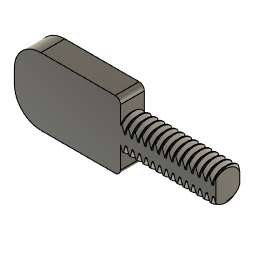
Printable 14-20 Bolt Handle v1 (Autodesk Fusion 360 design; units mm, degrees)
Autodesk Fusion 360 part; units mm, degrees
sketch "Sketch1" plane through (0, 0, 0) normal (1, 0, 0) x (0, 1, 0)
  circle A0 centre (0, 0) radius 3.175
  dimension "d1" = 6.35
  constraint coincident A0.centre origin
  measures "d1" diameter of A0
extrude "Extrude1" add sketch "Sketch1" along normal blind 18
sketch "Sketch2" plane through (0, 0, 0) normal (-1, 0, 0) x (0, -1, 0)
  circle A0 centre (0, 0) radius 3.175
  line L0 (5.5, 3.1754) -> (0, 6.3509)
  line L1 (0, 6.3509) -> (-5.5, 3.1754)
  line L2 (-5.5, 3.1754) -> (-5.5, -3.1754)
  line L3 (-5.5, -3.1754) -> (0, -6.3509)
  line L4 (0, -6.3509) -> (5.5, -3.1754)
  line L5 (5.5, -3.1754) -> (5.5, 3.1754)
  dimension "d4" = 11
  constraint coincident A0.centre origin
  constraint vertical L5
  measures "d4" distance of L2 L5
extrude "Extrude2" add sketch "Sketch2" along normal blind 4 contours A0 | L0 L1 L2 L3 L4 L5
thread "Thread1" "ANSI Unified Screw Threads 0.25 1/4-20 UNC 3A" major diameter 6.2484 minor diameter 4.8387 pitch 1.27 angle 60 modelled right hand crest width 0.1965 on face at (12, 3.1711, -0.1583) crest through (-0.3175, 3.1242, 0)
sketch "Sketch3" plane through (-4, 0, 0) normal (-1, 0, 0) x (0, -1, 0)
  line L0 (5.5, -3.1754) -> (5.5, 3.1754)
  line L1 (5.5, 3.1754) -> (0, 6.3509)
  line L2 (0, 6.3509) -> (-5.5, 3.1754)
  line L3 (-5.5, 3.1754) -> (-5.5, -3.1754)
  line L4 (-5.5, -3.1754) -> (0, -6.3509)
  line L5 (0, -6.3509) -> (5.5, -3.1754)
  line L6 (0, 0) -> (0, 21) construction
  line L7 (0, 0) -> (0, -19) construction
  line L8 (2.25, 5.0518) -> (2.25, -5.0518)
  line L9 (-2.25, 5.0518) -> (-2.25, -5.0518)
  dimension "d7" = 2.25
  dimension "d8" = 2.25
  constraint coincident L6.start L7.start
  constraint parallel L0 L6
  constraint parallel L6 L7
  constraint coincident L1 L8.start
  constraint coincident L5 L8.end
  constraint parallel L6 L8
  constraint coincident L2 L9.start
  constraint coincident L4 L9.end
  constraint parallel L7 L9
  measures "d7" distance of L6.start L9
  measures "d8" distance of L6 L8
extrude "Extrude3" cut sketch "Sketch3" against normal through all contours L0 L1 L5 L8 | L2 L3 L4 L9
sketch "Sketch4" plane through (0, -2.25, 0) normal (0, -1, 0) x (1, 0, 0)
  line L0 (0, -5.0518) -> (0, -1.2384)
  spline S0 degree 3 poles (0.3742, -2.1675) (0.295, -1.9904) (0.2175, -1.8092) (0.0949, -1.5007) (0.0458, -1.3702) (0, -1.2384) knots -0.136565 -0.136565 -0.136565 -0.136565 -0.077979 -0.077979 -0.036476 -0.036476 -0.036476 -0.036476
  line L1 (0.3742, -2.1675) -> (0.5707, -2.1675)
  spline S1 degree 3 poles (0.8988, -0.8892) (0.8665, -1.1289) (0.8148, -1.3659) (0.6999, -1.784) (0.6406, -1.969) (0.5748, -2.1561) (0.5728, -2.1618) (0.5707, -2.1675) knots -0.131697 -0.131697 -0.131697 -0.131697 -0.059487 -0.059487 -0.001818 -0.001818 0 0 0 0
  line L2 (0.8988, -0.8892) -> (1.1584, -0.8892)
  spline S2 degree 3 poles (1.6442, -2.1675) (1.565, -1.9904) (1.4875, -1.8092) (1.3222, -1.3933) (1.2345, -1.1492) (1.1614, -0.8997) (1.1599, -0.8945) (1.1584, -0.8892) knots -0.136565 -0.136565 -0.136565 -0.136565 -0.077979 -0.077979 -0.001638 -0.001638 0 0 0 0
  line L3 (1.6442, -2.1675) -> (1.8407, -2.1675)
  spline S3 degree 3 poles (2.1688, -0.8892) (2.1365, -1.1289) (2.0848, -1.3659) (1.9699, -1.784) (1.9106, -1.969) (1.8448, -2.1561) (1.8428, -2.1618) (1.8407, -2.1675) knots -0.131697 -0.131697 -0.131697 -0.131697 -0.059487 -0.059487 -0.001818 -0.001818 0 0 0 0
  line L4 (2.1688, -0.8892) -> (2.4284, -0.8892)
  spline S4 degree 3 poles (2.9142, -2.1675) (2.835, -1.9904) (2.7575, -1.8092) (2.5922, -1.3933) (2.5045, -1.1492) (2.4314, -0.8997) (2.4299, -0.8945) (2.4284, -0.8892) knots -0.136565 -0.136565 -0.136565 -0.136565 -0.077979 -0.077979 -0.001638 -0.001638 0 0 0 0
  line L5 (2.9142, -2.1675) -> (3.1107, -2.1675)
  spline S5 degree 3 poles (3.4388, -0.8892) (3.4065, -1.1289) (3.3548, -1.3659) (3.2399, -1.784) (3.1806, -1.969) (3.1148, -2.1561) (3.1128, -2.1618) (3.1107, -2.1675) knots -0.131697 -0.131697 -0.131697 -0.131697 -0.059487 -0.059487 -0.001818 -0.001818 0 0 0 0
  line L6 (3.4388, -0.8892) -> (3.6984, -0.8892)
  spline S6 degree 3 poles (4.1842, -2.1675) (4.105, -1.9904) (4.0275, -1.8092) (3.8622, -1.3933) (3.7745, -1.1492) (3.7014, -0.8997) (3.6999, -0.8945) (3.6984, -0.8892) knots -0.136565 -0.136565 -0.136565 -0.136565 -0.077979 -0.077979 -0.001638 -0.001638 0 0 0 0
  line L7 (4.1842, -2.1675) -> (4.3807, -2.1675)
  spline S7 degree 3 poles (4.7088, -0.8892) (4.6765, -1.1289) (4.6248, -1.3659) (4.5099, -1.784) (4.4506, -1.969) (4.3848, -2.1561) (4.3828, -2.1618) (4.3807, -2.1675) knots -0.131697 -0.131697 -0.131697 -0.131697 -0.059487 -0.059487 -0.001818 -0.001818 0 0 0 0
  line L8 (4.7088, -0.8892) -> (4.9684, -0.8892)
  spline S8 degree 3 poles (5.4542, -2.1675) (5.375, -1.9904) (5.2975, -1.8092) (5.1322, -1.3933) (5.0445, -1.1492) (4.9714, -0.8997) (4.9699, -0.8945) (4.9684, -0.8892) knots -0.136565 -0.136565 -0.136565 -0.136565 -0.077979 -0.077979 -0.001638 -0.001638 0 0 0 0
  line L9 (5.4542, -2.1675) -> (5.6507, -2.1675)
  spline S9 degree 3 poles (5.9788, -0.8892) (5.9465, -1.1289) (5.8948, -1.3659) (5.7799, -1.784) (5.7206, -1.969) (5.6548, -2.1561) (5.6528, -2.1618) (5.6507, -2.1675) knots -0.131697 -0.131697 -0.131697 -0.131697 -0.059487 -0.059487 -0.001818 -0.001818 0 0 0 0
  line L10 (5.9788, -0.8892) -> (6.2384, -0.8892)
  spline S10 degree 3 poles (6.7242, -2.1675) (6.645, -1.9904) (6.5675, -1.8092) (6.4022, -1.3933) (6.3145, -1.1492) (6.2414, -0.8997) (6.2399, -0.8945) (6.2384, -0.8892) knots -0.136565 -0.136565 -0.136565 -0.136565 -0.077979 -0.077979 -0.001638 -0.001638 0 0 0 0
  line L11 (6.7242, -2.1675) -> (6.9207, -2.1675)
  spline S11 degree 3 poles (7.2488, -0.8892) (7.2165, -1.1289) (7.1648, -1.3659) (7.0499, -1.784) (6.9906, -1.969) (6.9248, -2.1561) (6.9228, -2.1618) (6.9207, -2.1675) knots -0.131697 -0.131697 -0.131697 -0.131697 -0.059487 -0.059487 -0.001818 -0.001818 0 0 0 0
  line L12 (7.2488, -0.8892) -> (7.5084, -0.8892)
  spline S12 degree 3 poles (7.9942, -2.1675) (7.915, -1.9904) (7.8375, -1.8092) (7.6722, -1.3933) (7.5845, -1.1492) (7.5114, -0.8997) (7.5099, -0.8945) (7.5084, -0.8892) knots -0.136565 -0.136565 -0.136565 -0.136565 -0.077979 -0.077979 -0.001638 -0.001638 0 0 0 0
  line L13 (7.9942, -2.1675) -> (8.1907, -2.1675)
  spline S13 degree 3 poles (8.5188, -0.8892) (8.4865, -1.1289) (8.4348, -1.3659) (8.3199, -1.784) (8.2606, -1.969) (8.1948, -2.1561) (8.1928, -2.1618) (8.1907, -2.1675) knots -0.131697 -0.131697 -0.131697 -0.131697 -0.059487 -0.059487 -0.001818 -0.001818 0 0 0 0
  line L14 (8.5188, -0.8892) -> (8.7784, -0.8892)
  spline S14 degree 3 poles (9.2642, -2.1675) (9.185, -1.9904) (9.1075, -1.8092) (8.9422, -1.3933) (8.8545, -1.1492) (8.7814, -0.8997) (8.7799, -0.8945) (8.7784, -0.8892) knots -0.136565 -0.136565 -0.136565 -0.136565 -0.077979 -0.077979 -0.001638 -0.001638 0 0 0 0
  line L15 (9.2642, -2.1675) -> (9.4607, -2.1675)
  spline S15 degree 3 poles (9.7888, -0.8892) (9.7565, -1.1289) (9.7048, -1.3659) (9.5899, -1.784) (9.5306, -1.969) (9.4648, -2.1561) (9.4628, -2.1618) (9.4607, -2.1675) knots -0.131697 -0.131697 -0.131697 -0.131697 -0.059487 -0.059487 -0.001818 -0.001818 0 0 0 0
  line L16 (9.7888, -0.8892) -> (10.0484, -0.8892)
  spline S16 degree 3 poles (10.5342, -2.1675) (10.455, -1.9904) (10.3775, -1.8092) (10.2122, -1.3933) (10.1245, -1.1492) (10.0514, -0.8997) (10.0499, -0.8945) (10.0484, -0.8892) knots -0.136565 -0.136565 -0.136565 -0.136565 -0.077979 -0.077979 -0.001638 -0.001638 0 0 0 0
  line L17 (10.5342, -2.1675) -> (10.7307, -2.1675)
  spline S17 degree 3 poles (11.0588, -0.8892) (11.0265, -1.1289) (10.9748, -1.3659) (10.8599, -1.784) (10.8006, -1.969) (10.7348, -2.1561) (10.7328, -2.1618) (10.7307, -2.1675) knots -0.131697 -0.131697 -0.131697 -0.131697 -0.059487 -0.059487 -0.001818 -0.001818 0 0 0 0
  line L18 (11.0588, -0.8892) -> (11.3184, -0.8892)
  spline S18 degree 3 poles (11.8042, -2.1675) (11.725, -1.9904) (11.6475, -1.8092) (11.4822, -1.3933) (11.3945, -1.1492) (11.3214, -0.8997) (11.3199, -0.8945) (11.3184, -0.8892) knots -0.136565 -0.136565 -0.136565 -0.136565 -0.077979 -0.077979 -0.001638 -0.001638 0 0 0 0
  line L19 (11.8042, -2.1675) -> (12.0007, -2.1675)
  spline S19 degree 3 poles (12.3288, -0.8892) (12.2965, -1.1289) (12.2448, -1.3659) (12.1299, -1.784) (12.0706, -1.969) (12.0048, -2.1561) (12.0028, -2.1618) (12.0007, -2.1675) knots -0.131697 -0.131697 -0.131697 -0.131697 -0.059487 -0.059487 -0.001818 -0.001818 0 0 0 0
  line L20 (12.3288, -0.8892) -> (12.5884, -0.8892)
  spline S20 degree 3 poles (13.0742, -2.1675) (12.995, -1.9904) (12.9175, -1.8092) (12.7522, -1.3933) (12.6645, -1.1492) (12.5914, -0.8997) (12.5899, -0.8945) (12.5884, -0.8892) knots -0.136565 -0.136565 -0.136565 -0.136565 -0.077979 -0.077979 -0.001638 -0.001638 0 0 0 0
  line L21 (13.0742, -2.1675) -> (13.2707, -2.1675)
  spline S21 degree 3 poles (13.5988, -0.8892) (13.5665, -1.1289) (13.5148, -1.3659) (13.3999, -1.784) (13.3406, -1.969) (13.2748, -2.1561) (13.2728, -2.1618) (13.2707, -2.1675) knots -0.131697 -0.131697 -0.131697 -0.131697 -0.059487 -0.059487 -0.001818 -0.001818 0 0 0 0
  line L22 (13.5988, -0.8892) -> (13.8584, -0.8892)
  spline S22 degree 3 poles (14.3442, -2.1675) (14.265, -1.9904) (14.1875, -1.8092) (14.0222, -1.3933) (13.9345, -1.1492) (13.8614, -0.8997) (13.8599, -0.8945) (13.8584, -0.8892) knots -0.136565 -0.136565 -0.136565 -0.136565 -0.077979 -0.077979 -0.001638 -0.001638 0 0 0 0
  line L23 (14.3442, -2.1675) -> (14.5407, -2.1675)
  spline S23 degree 3 poles (14.8688, -0.8892) (14.8365, -1.1289) (14.7848, -1.3659) (14.6699, -1.784) (14.6106, -1.969) (14.5448, -2.1561) (14.5428, -2.1618) (14.5407, -2.1675) knots -0.131697 -0.131697 -0.131697 -0.131697 -0.059487 -0.059487 -0.001818 -0.001818 0 0 0 0
  line L24 (14.8688, -0.8892) -> (15.1284, -0.8892)
  spline S24 degree 3 poles (15.6142, -2.1675) (15.535, -1.9904) (15.4575, -1.8092) (15.2922, -1.3933) (15.2045, -1.1492) (15.1314, -0.8997) (15.1299, -0.8945) (15.1284, -0.8892) knots -0.136565 -0.136565 -0.136565 -0.136565 -0.077979 -0.077979 -0.001638 -0.001638 0 0 0 0
  line L25 (15.6142, -2.1675) -> (15.8107, -2.1675)
  spline S25 degree 3 poles (16.1388, -0.8892) (16.1065, -1.1289) (16.0548, -1.3659) (15.9399, -1.784) (15.8806, -1.969) (15.8148, -2.1561) (15.8128, -2.1618) (15.8107, -2.1675) knots -0.131697 -0.131697 -0.131697 -0.131697 -0.059487 -0.059487 -0.001818 -0.001818 0 0 0 0
  line L26 (16.1388, -0.8892) -> (16.3984, -0.8892)
  spline S26 degree 3 poles (16.8842, -2.1675) (16.805, -1.9904) (16.7275, -1.8092) (16.5622, -1.3933) (16.4745, -1.1492) (16.4014, -0.8997) (16.3999, -0.8945) (16.3984, -0.8892) knots -0.136565 -0.136565 -0.136565 -0.136565 -0.077979 -0.077979 -0.001638 -0.001638 0 0 0 0
  line L27 (16.8842, -2.1675) -> (17.0807, -2.1675)
  spline S27 degree 3 poles (17.4088, -0.8892) (17.3765, -1.1289) (17.3248, -1.3659) (17.2099, -1.784) (17.1506, -1.969) (17.0848, -2.1561) (17.0828, -2.1618) (17.0807, -2.1675) knots -0.131697 -0.131697 -0.131697 -0.131697 -0.059487 -0.059487 -0.001818 -0.001818 0 0 0 0
  line L28 (17.4088, -0.8892) -> (17.6684, -0.8892)
  spline S28 degree 3 poles (18, -1.811) (17.9747, -1.7502) (17.9499, -1.6894) (17.8322, -1.3933) (17.7445, -1.1492) (17.6714, -0.8997) (17.6699, -0.8945) (17.6684, -0.8892) knots -0.097692 -0.097692 -0.097692 -0.097692 -0.077979 -0.077979 -0.001638 -0.001638 0 0 0 0
  line L29 (18, -1.811) -> (18, 2.1675)
  line L30 (18, 2.1675) -> (17.8443, 2.1675)
  spline S29 degree 3 poles (17.5162, 0.8892) (17.5494, 1.1359) (17.6033, 1.3798) (17.721, 1.8032) (17.7804, 1.9872) (17.8443, 2.1675) knots -0.13167 -0.13167 -0.13167 -0.13167 -0.057372 -0.057372 0 0 0 0
  line L31 (17.5162, 0.8892) -> (17.2566, 0.8892)
  spline S30 degree 3 poles (16.7708, 2.1675) (16.8514, 1.9872) (16.9303, 1.8026) (17.0972, 1.3816) (17.1853, 1.1355) (17.2566, 0.8892) knots -0.136566 -0.136566 -0.136566 -0.136566 -0.076908 -0.076908 0 0 0 0
  line L32 (16.7708, 2.1675) -> (16.5743, 2.1675)
  spline S31 degree 3 poles (16.2462, 0.8892) (16.2794, 1.1359) (16.3333, 1.3798) (16.451, 1.8032) (16.5104, 1.9872) (16.5743, 2.1675) knots -0.13167 -0.13167 -0.13167 -0.13167 -0.057372 -0.057372 0 0 0 0
  line L33 (16.2462, 0.8892) -> (15.9866, 0.8892)
  spline S32 degree 3 poles (15.5008, 2.1675) (15.5814, 1.9872) (15.6603, 1.8026) (15.8272, 1.3816) (15.9153, 1.1355) (15.9866, 0.8892) knots -0.136566 -0.136566 -0.136566 -0.136566 -0.076908 -0.076908 0 0 0 0
  line L34 (15.5008, 2.1675) -> (15.3043, 2.1675)
  spline S33 degree 3 poles (14.9762, 0.8892) (15.0094, 1.1359) (15.0633, 1.3798) (15.181, 1.8032) (15.2404, 1.9872) (15.3043, 2.1675) knots -0.13167 -0.13167 -0.13167 -0.13167 -0.057372 -0.057372 0 0 0 0
  line L35 (14.9762, 0.8892) -> (14.7166, 0.8892)
  spline S34 degree 3 poles (14.2308, 2.1675) (14.3114, 1.9872) (14.3903, 1.8026) (14.5572, 1.3816) (14.6453, 1.1355) (14.7166, 0.8892) knots -0.136566 -0.136566 -0.136566 -0.136566 -0.076908 -0.076908 0 0 0 0
  line L36 (14.2308, 2.1675) -> (14.0343, 2.1675)
  spline S35 degree 3 poles (13.7062, 0.8892) (13.7394, 1.1359) (13.7933, 1.3798) (13.911, 1.8032) (13.9704, 1.9872) (14.0343, 2.1675) knots -0.13167 -0.13167 -0.13167 -0.13167 -0.057372 -0.057372 0 0 0 0
  line L37 (13.7062, 0.8892) -> (13.4466, 0.8892)
  spline S36 degree 3 poles (12.9608, 2.1675) (13.0414, 1.9872) (13.1203, 1.8026) (13.2872, 1.3816) (13.3753, 1.1355) (13.4466, 0.8892) knots -0.136566 -0.136566 -0.136566 -0.136566 -0.076908 -0.076908 0 0 0 0
  line L38 (12.9608, 2.1675) -> (12.7643, 2.1675)
  spline S37 degree 3 poles (12.4362, 0.8892) (12.4694, 1.1359) (12.5233, 1.3798) (12.641, 1.8032) (12.7004, 1.9872) (12.7643, 2.1675) knots -0.13167 -0.13167 -0.13167 -0.13167 -0.057372 -0.057372 0 0 0 0
  line L39 (12.4362, 0.8892) -> (12.1766, 0.8892)
  spline S38 degree 3 poles (11.6908, 2.1675) (11.7714, 1.9872) (11.8503, 1.8026) (12.0172, 1.3816) (12.1053, 1.1355) (12.1766, 0.8892) knots -0.136566 -0.136566 -0.136566 -0.136566 -0.076908 -0.076908 0 0 0 0
  line L40 (11.6908, 2.1675) -> (11.4943, 2.1675)
  spline S39 degree 3 poles (11.1662, 0.8892) (11.1994, 1.1359) (11.2533, 1.3798) (11.371, 1.8032) (11.4304, 1.9872) (11.4943, 2.1675) knots -0.13167 -0.13167 -0.13167 -0.13167 -0.057372 -0.057372 0 0 0 0
  line L41 (11.1662, 0.8892) -> (10.9066, 0.8892)
  spline S40 degree 3 poles (10.4208, 2.1675) (10.5014, 1.9872) (10.5803, 1.8026) (10.7472, 1.3816) (10.8353, 1.1355) (10.9066, 0.8892) knots -0.136566 -0.136566 -0.136566 -0.136566 -0.076908 -0.076908 0 0 0 0
  line L42 (10.4208, 2.1675) -> (10.2243, 2.1675)
  spline S41 degree 3 poles (9.8962, 0.8892) (9.9294, 1.1359) (9.9833, 1.3798) (10.101, 1.8032) (10.1604, 1.9872) (10.2243, 2.1675) knots -0.13167 -0.13167 -0.13167 -0.13167 -0.057372 -0.057372 0 0 0 0
  line L43 (9.8962, 0.8892) -> (9.6366, 0.8892)
  spline S42 degree 3 poles (9.1508, 2.1675) (9.2314, 1.9872) (9.3103, 1.8026) (9.4772, 1.3816) (9.5653, 1.1355) (9.6366, 0.8892) knots -0.136566 -0.136566 -0.136566 -0.136566 -0.076908 -0.076908 0 0 0 0
  line L44 (9.1508, 2.1675) -> (8.9543, 2.1675)
  spline S43 degree 3 poles (8.6262, 0.8892) (8.6594, 1.1359) (8.7133, 1.3798) (8.831, 1.8032) (8.8904, 1.9872) (8.9543, 2.1675) knots -0.13167 -0.13167 -0.13167 -0.13167 -0.057372 -0.057372 0 0 0 0
  line L45 (8.6262, 0.8892) -> (8.3666, 0.8892)
  spline S44 degree 3 poles (7.8808, 2.1675) (7.9614, 1.9872) (8.0403, 1.8026) (8.2072, 1.3816) (8.2953, 1.1355) (8.3666, 0.8892) knots -0.136566 -0.136566 -0.136566 -0.136566 -0.076908 -0.076908 0 0 0 0
  line L46 (7.8808, 2.1675) -> (7.6843, 2.1675)
  spline S45 degree 3 poles (7.3562, 0.8892) (7.3894, 1.1359) (7.4433, 1.3798) (7.561, 1.8032) (7.6204, 1.9872) (7.6843, 2.1675) knots -0.13167 -0.13167 -0.13167 -0.13167 -0.057372 -0.057372 0 0 0 0
  line L47 (7.3562, 0.8892) -> (7.0966, 0.8892)
  spline S46 degree 3 poles (6.6108, 2.1675) (6.6914, 1.9872) (6.7703, 1.8026) (6.9372, 1.3816) (7.0253, 1.1355) (7.0966, 0.8892) knots -0.136566 -0.136566 -0.136566 -0.136566 -0.076908 -0.076908 0 0 0 0
  line L48 (6.6108, 2.1675) -> (6.4143, 2.1675)
  spline S47 degree 3 poles (6.0862, 0.8892) (6.1194, 1.1359) (6.1733, 1.3798) (6.291, 1.8032) (6.3504, 1.9872) (6.4143, 2.1675) knots -0.13167 -0.13167 -0.13167 -0.13167 -0.057372 -0.057372 0 0 0 0
  line L49 (6.0862, 0.8892) -> (5.8266, 0.8892)
  spline S48 degree 3 poles (5.3408, 2.1675) (5.4214, 1.9872) (5.5003, 1.8026) (5.6672, 1.3816) (5.7553, 1.1355) (5.8266, 0.8892) knots -0.136566 -0.136566 -0.136566 -0.136566 -0.076908 -0.076908 0 0 0 0
  line L50 (5.3408, 2.1675) -> (5.1443, 2.1675)
  spline S49 degree 3 poles (4.8162, 0.8892) (4.8494, 1.1359) (4.9033, 1.3798) (5.021, 1.8032) (5.0804, 1.9872) (5.1443, 2.1675) knots -0.13167 -0.13167 -0.13167 -0.13167 -0.057372 -0.057372 0 0 0 0
  line L51 (4.8162, 0.8892) -> (4.5566, 0.8892)
  spline S50 degree 3 poles (4.0708, 2.1675) (4.1514, 1.9872) (4.2303, 1.8026) (4.3972, 1.3816) (4.4853, 1.1355) (4.5566, 0.8892) knots -0.136566 -0.136566 -0.136566 -0.136566 -0.076908 -0.076908 0 0 0 0
  line L52 (4.0708, 2.1675) -> (3.8743, 2.1675)
  spline S51 degree 3 poles (3.5462, 0.8892) (3.5794, 1.1359) (3.6333, 1.3798) (3.751, 1.8032) (3.8104, 1.9872) (3.8743, 2.1675) knots -0.13167 -0.13167 -0.13167 -0.13167 -0.057372 -0.057372 0 0 0 0
  line L53 (3.5462, 0.8892) -> (3.2866, 0.8892)
  spline S52 degree 3 poles (2.8008, 2.1675) (2.8814, 1.9872) (2.9603, 1.8026) (3.1272, 1.3816) (3.2153, 1.1355) (3.2866, 0.8892) knots -0.136566 -0.136566 -0.136566 -0.136566 -0.076908 -0.076908 0 0 0 0
  line L54 (2.8008, 2.1675) -> (2.6043, 2.1675)
  spline S53 degree 3 poles (2.2762, 0.8892) (2.3094, 1.1359) (2.3633, 1.3798) (2.481, 1.8032) (2.5404, 1.9872) (2.6043, 2.1675) knots -0.13167 -0.13167 -0.13167 -0.13167 -0.057372 -0.057372 0 0 0 0
  line L55 (2.2762, 0.8892) -> (2.0166, 0.8892)
  spline S54 degree 3 poles (1.5308, 2.1675) (1.6114, 1.9872) (1.6903, 1.8026) (1.8572, 1.3816) (1.9453, 1.1355) (2.0166, 0.8892) knots -0.136566 -0.136566 -0.136566 -0.136566 -0.076908 -0.076908 0 0 0 0
  line L56 (1.5308, 2.1675) -> (1.3343, 2.1675)
  spline S55 degree 3 poles (1.0062, 0.8892) (1.0394, 1.1359) (1.0933, 1.3798) (1.211, 1.8032) (1.2704, 1.9872) (1.3343, 2.1675) knots -0.13167 -0.13167 -0.13167 -0.13167 -0.057372 -0.057372 0 0 0 0
  line L57 (1.0062, 0.8892) -> (0.7466, 0.8892)
  spline S56 degree 3 poles (0.2608, 2.1675) (0.3414, 1.9872) (0.4203, 1.8026) (0.5872, 1.3816) (0.6753, 1.1355) (0.7466, 0.8892) knots -0.136566 -0.136566 -0.136566 -0.136566 -0.076908 -0.076908 0 0 0 0
  line L58 (0.2608, 2.1675) -> (0.0643, 2.1675)
  spline S57 degree 3 poles (0, 1.9799) (0.0208, 2.0428) (0.0423, 2.1054) (0.0643, 2.1675) knots -0.019771 -0.019771 -0.019771 -0.019771 0 0 0 0
  line L59 (0, 1.9799) -> (0, 5.0518)
  line L60 (0, 5.0518) -> (-4, 5.0518)
  line L61 (-4, 5.0518) -> (-4, -5.0518)
  line L62 (-4, -5.0518) -> (0, -5.0518)
  line L63 (0, 0) -> (-20, 0)
  line L64 (-20, 0) -> (-20, 6.3509)
  line L65 (-20, 6.3509) -> (0, 6.3509)
  line L66 (0, 6.3509) -> (0, 0)
  line L67 (0, 0) -> (-20, 0)
  line L68 (-20, 0) -> (-20, -6.3509)
  line L69 (-20, -6.3509) -> (0, -6.3509)
  line L70 (0, -6.3509) -> (0, 0)
  point P0 (0, -6.3509)
  point P1 (0, 6.3509)
  dimension "d11" = 20
  constraint horizontal L63
  constraint vertical L64
  constraint horizontal L65
  constraint vertical L66
  constraint coincident L63.start L66.end
  constraint horizontal L67
  constraint vertical L68
  constraint horizontal L69
  constraint vertical L70
  constraint coincident L69 P0
  constraint coincident P1 L65.end
  constraint collinear L64 L68
  measures "d11" distance of L64.end P1
extrude "Extrude4" add sketch "Sketch4" against normal up to surface (4.5 mm away) contours L0 L61 L62 L63 L67 L70 | L61 L62 L63 L67 L68 L69 L70 | L59 L60 L61 L63 L66 L67 | L60 L61 L63 L64 L65 L66 L67
fillet "Fillet2" radius 1 2 edges at (0, 0, 6.3509) (0, 0, -6.3509)
fillet "Fillet3" radius 5 2 edges at (-20, 0, -6.3509) (-20, 0, 6.3509)
